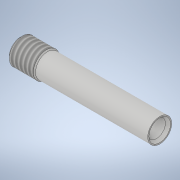
# Autodesk Inventor part: MINI-heatbreak
Saved by Autodesk Inventor 2021 (Build 250183000, 183)
## iProperties
Created: 2019-09-24
Material: Všeobecné
Document SubType Name: Modeling
Density: 1 g/cm^3
Appearance: Výchozí
Project: ORIGINAL PRUSA MINI
Authority: Ing. Robert Turinský
Company: Prusa Development a.s.
Author: Ing. Robert Turinský
Title: MINI-heatbreak
Revision Number: R4
Autodesk Inventor part; units mm, degrees
ref_plane "YZ Plane" through (0, 0, 0) normal (1, 0, 0) x (0, 1, 0)
ref_plane "XZ Plane" through (0, 0, 0) normal (0, 1, 0) x (-1, 0, 0)
ref_plane "XY Plane" through (0, 0, 0) normal (0, 0, 1) x (1, 0, 0)
sketch "Náčrt1" plane through (0, 0, 0) normal (0, 0, 1) x (1, 0, 0)
  line L0 (0, -3.6) -> (0, 0.6) projected
  line L1 (-6.4, 0) -> (38.4, 0) projected
  line L2 (0, -1) -> (6, -1)
  line L3 (32, -2.75) -> (6.25, -2.75)
  line L4 (6.25, -2.75) -> (6, -3)
  line L5 (6, -3) -> (0.5, -3)
  line L6 (0.5, -3) -> (0, -2.5)
  line L7 (0, -2.5) -> (0, -1)
  line L8 (32, -2.75) -> (32, -2.05)
  line L9 (6, -1) -> (6.6309, -2.05)
  line L10 (6.6309, -2.05) -> (32, -2.05)
  point P0 (0, 0)
  dimension "d0" = 2
  dimension "d1" = 5.5
  dimension "d3" = 6
  dimension "d4" = 45
  dimension "d5" = 6
  dimension "d6" = 0.5
  dimension "d7" = 90
  dimension "d16" = 4.1
  dimension "d17" = 59
  dimension "d18" = 26
  dimension "d19" = 6
  constraints: 18 end point, 2 perpendicular, 2 point on line, 1 collinear, 1 horizontal, 1 parallel
  measures "d0" diameter of L2 L1
  measures "d1" diameter of L3 L1
  measures "d3" diameter of L5 L1
  measures "d4" angle of L0 L6
  measures "d5" distance from line of L0 L4.end
  measures "d6" horizontal distance of L5.end L6.end
  measures "d7" angle of L3 L8
  measures "d16" diameter of L10 L1
  measures "d17" angle of L1 L9
  measures "d18" horizontal distance of L4.end L3.start
  measures "d19" distance from line of L0 L2.end
revolve "Rotace1" add sketch "Náčrt1" angle 360 about axis through (-10, 0, 0) along (1, 0, 0)
thread "Závit1" size "M6x1" class "6g" standard "ANSI Metric M Profile" full length
chamfer "Zkosení1" distance 0.75 angle 30 1 edges at (32, 2.05, 0) measured on face at (15.0873, -2.0235, 0.3288)
